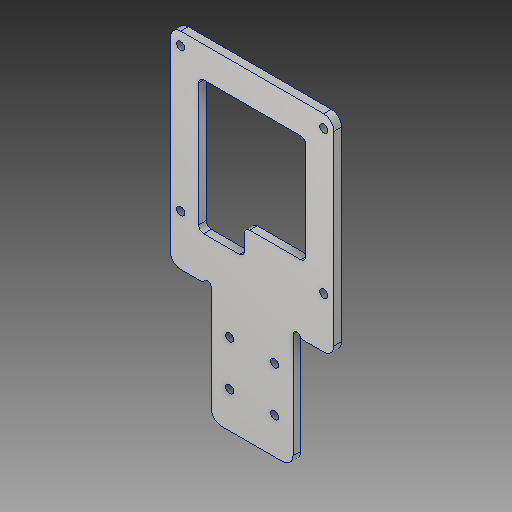
# Autodesk Inventor part: 手先カメラ
Saved by Autodesk Inventor 2017 (Build 210142000, 142)
## iProperties
Created: 2016-11-26
Part Number: 手先カメラ
Material: アルミニウム 6061
Document SubType Name: Modeling
Designer: NN
Density: 2.7 g/cm^3
Appearance: アルミニウム - フラット
Mass: 4.6771 g
Surface Area: 28.0851 cm^2
Volume: 1.73226 cm^3
Author: NN
Autodesk Inventor part; units mm, degrees
ref_plane "YZ Plane" through (0, 0, 0) normal (1, 0, 0) x (0, 1, 0)
ref_plane "XZ Plane" through (0, 0, 0) normal (0, 1, 0) x (-1, 0, 0)
ref_plane "XY Plane" through (0, 0, 0) normal (0, 0, 1) x (1, 0, 0)
sketch "スケッチ1" plane through (0, 0, 0) normal (0, 0, 1) x (1, 0, 0)
  line L0 (0, 0) -> (32, 0)
  line L1 (32, 0) -> (32, 63)
  line L2 (32, 63) -> (0, 63)
  line L3 (0, 63) -> (0, 0)
  dimension "d0" = 32
  dimension "d1" = 63
  constraints: 8 end point, 2 parallel, 1 horizontal, 1 perpendicular
  measures "d0" distance of L1.end L2.end
  measures "d1" distance between parallel lines of L0 L2
extrude "押し出し1" add sketch "スケッチ1" along normal blind 1.5
sketch "スケッチ2" plane through (0, 0, 1.5) normal (0, 0, 1) x (1, 0, 0)
  line L0 (2, 60.5) -> (30, 60.5)
  line L1 (30, 60.5) -> (30, 32.5)
  line L2 (30, 32.5) -> (2, 32.5)
  line L3 (2, 32.5) -> (2, 60.5)
  line L4 (32, 63) -> (0, 63) projected
  line L5 (16, 63) -> (16, 60.5)
  point P0 (0, 0)
  dimension "d4" = 28
  dimension "d5" = 28
  dimension "d6" = 2.5
  constraints: 10 end point, 2 midpoint, 2 parallel, 2 perpendicular, 1 horizontal
  measures "d4" distance of L0.start L0.end
  measures "d5" distance of L2.end L0.start
  measures "d6" distance between parallel lines of L4 L0
hole "穴1" at (30, 60.5, 1.5) at (2, 60.5, 1.5) at (30, 32.5, 1.5) at (2, 32.5, 1.5) direction (0, 0, -1) diameter 1.567 end through all thread size "M2x0.4" class "6H" standard "ISO Metric profile"
sketch "スケッチ3" plane through (0, 0, 1.5) normal (0, 0, 1) x (1, 0, 0)
  circle A0 centre (30, 32.5) radius 0.7835 projected
  circle A1 centre (30, 60.5) radius 0.7835 projected
  circle A2 centre (2, 60.5) radius 0.7835 projected
  circle A3 centre (2, 32.5) radius 0.7835 projected
  line L0 (0, 0) -> (32, 0) projected
  line L1 (32, 0) -> (32, 63) projected
  line L2 (32, 63) -> (0, 63) projected
  line L3 (0, 63) -> (0, 0) projected
  line L4 (0, 0) -> (8, 0)
  line L5 (8, 0) -> (8, 22.6)
  line L6 (8, 22.6) -> (0, 22.6)
  line L7 (0, 22.6) -> (0, 0)
  line L8 (0, 0) -> (32, 0) projected
  line L9 (16, 0) -> (16, 3.4564)
  line L10 (32, 0) -> (24, 0)
  line L11 (24, 0) -> (24, 22.6)
  line L12 (24, 22.6) -> (32, 22.6)
  line L13 (32, 22.6) -> (32, 0)
  dimension "d14" = 22.6
  dimension "d15" = 16
  constraints: 18 end point, 5 symmetric about line, 2 parallel, 1 horizontal, 1 midpoint, 1 perpendicular, 1 vertical
  measures "d14" distance between parallel lines of L0 L6
  measures "d15" distance between parallel lines of L11 L5
extrude "押し出し2" cut sketch "スケッチ3" against normal through all contours L3 L6 L5 L0 | L11 L12 L1 L0
sketch "スケッチ4" plane through (0, 0, 1.5) normal (0, 0, 1) x (1, 0, 0)
  line L0 (8, 22.6) -> (8, 0) projected
  line L1 (8, 0) -> (24, 0) projected
  line L2 (24, 0) -> (24, 22.6) projected
  line L3 (24, 22.6) -> (32, 22.6) projected
  line L4 (32, 22.6) -> (32, 63) projected
  line L5 (32, 63) -> (0, 63) projected
  line L6 (0, 63) -> (0, 22.6) projected
  line L7 (0, 22.6) -> (8, 22.6) projected
  circle A0 centre (30, 32.5) radius 0.7835 projected
  circle A1 centre (30, 60.5) radius 0.7835 projected
  circle A2 centre (2, 60.5) radius 0.7835 projected
  circle A3 centre (2, 32.5) radius 0.7835 projected
  line L8 (11.6, 15.9) -> (20.4, 15.9)
  line L9 (20.4, 15.9) -> (20.4, 7.1)
  line L10 (20.4, 7.1) -> (11.6, 7.1)
  line L11 (11.6, 7.1) -> (11.6, 15.9)
  line L12 (8, 0) -> (24, 0) projected
  line L13 (16, 0) -> (16, 7.1)
  line L14 (24, 0) -> (24, 22.6) projected
  line L15 (8, 0) -> (24, 0) projected
  point P0 (0, 0)
  dimension "d18" = 8.8
  dimension "d19" = 8.8
  dimension "d27" = 6.7
  constraints: 10 end point, 2 midpoint, 2 parallel, 2 perpendicular, 1 horizontal
  measures "d18" distance of L9.end L10.end
  measures "d19" distance of L8.end L9.end
  measures "d27" distance between parallel lines of L3 L8
hole "穴2" at (20.4, 15.9, 1.5) at (20.4, 7.1, 1.5) at (11.6, 7.1, 1.5) at (11.6, 15.9, 1.5) direction (0, 0, -1) diameter 1.567 end through all thread size "M2x0.4" class "6H" standard "ISO Metric profile"
sketch "スケッチ5" plane through (0, 0, 0) normal (0, 0, -1) x (-1, 0, 0)
  line L0 (-6, 34.6) -> (-14, 34.6) projected
  line L1 (-14, 34.6) -> (-14, 31.4) projected
  line L2 (-14, 31.4) -> (-6, 31.4) projected
  line L3 (-6, 31.4) -> (-6, 34.6) projected
  line L4 (-14.5, 35.1) -> (-5.5, 35.1)
  line L5 (-5.5, 35.1) -> (-5.5, 30.9)
  line L6 (-5.5, 30.9) -> (-14.5, 30.9)
  line L7 (-14.5, 30.9) -> (-14.5, 35.1)
  point P0 (0, 0)
  dimension "d28" = 0.5
  constraints: 8 end point, 3 other
  measures "d28" distance between parallel lines of L4 L0
extrude "押し出し3" cut sketch "スケッチ5" against normal through all contours L3 L2 L1 L0 | L4 L5 L6 L7
fillet "フィレット1" radius 2 6 edges at (32, 63, 0.75) (0, 63, 0.75) (0, 22.6, 0.75) (32, 22.6, 0.75) (8, 0, 0.75) (24, 0, 0.75)
sketch "スケッチ6" plane through (0, 0, 1.5) normal (0, 0, 1) x (1, 0, 0)
  line L0 (14.5, 35.1) -> (14.5, 30.9) projected
  line L1 (14.5, 30.9) -> (5.5, 30.9) projected
  line L2 (5.5, 30.9) -> (5.5, 35.1) projected
  line L3 (5.5, 35.1) -> (14.5, 35.1) projected
  circle A0 centre (11.6, 7.1) radius 0.7835 projected
  circle A1 centre (20.4, 15.9) radius 0.7835 projected
  circle A2 centre (20.4, 7.1) radius 0.7835 projected
  circle A3 centre (11.6, 15.9) radius 0.7835 projected
  arc A4 (22, 0) -> (24, 2) centre (22, 2) ccw projected
  line L4 (24, 2) -> (24, 22.6) projected
  line L5 (24, 22.6) -> (30, 22.6) projected
  arc A5 (30, 22.6) -> (32, 24.6) centre (30, 24.6) ccw projected
  line L6 (32, 24.6) -> (32, 61) projected
  arc A6 (32, 61) -> (30, 63) centre (30, 61) ccw projected
  line L7 (30, 63) -> (2, 63) projected
  arc A7 (2, 63) -> (0, 61) centre (2, 61) ccw projected
  line L8 (0, 61) -> (0, 24.6) projected
  arc A8 (0, 24.6) -> (2, 22.6) centre (2, 24.6) ccw projected
  line L9 (2, 22.6) -> (8, 22.6) projected
  line L10 (8, 22.6) -> (8, 2) projected
  arc A9 (8, 2) -> (10, 0) centre (10, 2) ccw projected
  line L11 (10, 0) -> (22, 0) projected
  circle A10 centre (30, 32.5) radius 0.7835 projected
  circle A11 centre (30, 60.5) radius 0.7835 projected
  circle A12 centre (2, 60.5) radius 0.7835 projected
  circle A13 centre (2, 32.5) radius 0.7835 projected
  line L12 (8, 22.6) -> (2, 22.6) projected
  circle A14 centre (7.25, 22.6) radius 0.75
  line L13 (30, 22.6) -> (24, 22.6) projected
  circle A15 centre (24.75, 22.6) radius 0.75
  line L14 (8, 22.6) -> (8, 2) projected
  line L15 (24, 2) -> (24, 22.6) projected
  point P0 (0, 0)
  dimension "d34" = 1.5
  dimension "d35" = 1.5
  constraints: 2 centre point, 2 point on line, 2 tangent
  measures "d34" diameter of A14
  measures "d35" diameter of A15
extrude "押し出し4" cut sketch "スケッチ6" against normal through all contours A15 L5 | L5 A15 | A14 L9 | L9 A14
fillet "フィレット2" radius 1 4 edges at (8, 22.6, 0.75) (6.5, 22.6, 0.75) (25.5, 22.6, 0.75) (24, 22.6, 0.75)
sketch "スケッチ7" plane through (0, 0, 1.5) normal (0, 0, 1) x (1, 0, 0)
  arc A0 (25.3655, 23.0286) -> (26.1861, 22.6) centre (26.1861, 23.6) ccw projected
  line L0 (26.1861, 22.6) -> (30, 22.6) projected
  arc A1 (30, 22.6) -> (32, 24.6) centre (30, 24.6) ccw projected
  line L1 (32, 24.6) -> (32, 61) projected
  arc A2 (32, 61) -> (30, 63) centre (30, 61) ccw projected
  line L2 (30, 63) -> (2, 63) projected
  arc A3 (2, 63) -> (0, 61) centre (2, 61) ccw projected
  line L3 (0, 61) -> (0, 24.6) projected
  arc A4 (0, 24.6) -> (2, 22.6) centre (2, 24.6) ccw projected
  line L4 (2, 22.6) -> (5.8139, 22.6) projected
  arc A5 (5.8139, 22.6) -> (6.6345, 23.0286) centre (5.8139, 23.6) ccw projected
  arc A6 (8, 22.6) -> (6.6345, 23.0286) centre (7.25, 22.6) ccw projected
  line L5 (8, 22.6) -> (8, 2) projected
  arc A7 (8, 2) -> (10, 0) centre (10, 2) ccw projected
  line L6 (10, 0) -> (22, 0) projected
  arc A8 (22, 0) -> (24, 2) centre (22, 2) ccw projected
  line L7 (24, 2) -> (24, 22.6) projected
  arc A9 (25.3655, 23.0286) -> (24, 22.6) centre (24.75, 22.6) ccw projected
  line L8 (14.5, 35.1) -> (14.5, 30.9) projected
  line L9 (14.5, 30.9) -> (5.5, 30.9) projected
  line L10 (5.5, 30.9) -> (5.5, 35.1) projected
  line L11 (5.5, 35.1) -> (14.5, 35.1) projected
  circle A10 centre (11.6, 7.1) radius 0.7835 projected
  circle A11 centre (20.4, 15.9) radius 0.7835 projected
  circle A12 centre (20.4, 7.1) radius 0.7835 projected
  circle A13 centre (11.6, 15.9) radius 0.7835 projected
  circle A14 centre (30, 32.5) radius 0.7835 projected
  circle A15 centre (30, 60.5) radius 0.7835 projected
  circle A16 centre (2, 60.5) radius 0.7835 projected
  circle A17 centre (2, 32.5) radius 0.7835 projected
  circle A18 centre (2, 60.5) radius 0.7835 projected
  line L12 (2, 60.5) -> (30, 60.5)
  line L13 (30, 60.5) -> (30, 32.5)
  line L14 (30, 32.5) -> (2, 32.5)
  line L15 (2, 32.5) -> (2, 60.5)
  line L16 (26.5, 57) -> (5.5, 57)
  line L17 (5.5, 57) -> (5.5, 36)
  line L18 (5.5, 36) -> (26.5, 36)
  line L19 (26.5, 36) -> (26.5, 57)
  point P0 (0, 0)
  dimension "d38" = 21
  constraints: 16 end point, 4 parallel, 2 perpendicular, 1 horizontal, 3 other
  measures "d38" distance between parallel lines of L19 L17
extrude "押し出し5" cut sketch "スケッチ7" against normal through all contours L19 L18 L17 L16
sketch "スケッチ8" plane through (0, 0, 1.5) normal (0, 0, 1) x (1, 0, 0)
  line L0 (5.5, 36) -> (5.5, 57) projected
  line L1 (5.5, 57) -> (26.5, 57) projected
  line L2 (26.5, 57) -> (26.5, 36) projected
  line L3 (26.5, 36) -> (5.5, 36) projected
  arc A0 (25.3655, 23.0286) -> (26.1861, 22.6) centre (26.1861, 23.6) ccw projected
  line L4 (26.1861, 22.6) -> (30, 22.6) projected
  arc A1 (30, 22.6) -> (32, 24.6) centre (30, 24.6) ccw projected
  line L5 (32, 24.6) -> (32, 61) projected
  arc A2 (32, 61) -> (30, 63) centre (30, 61) ccw projected
  line L6 (30, 63) -> (2, 63) projected
  arc A3 (2, 63) -> (0, 61) centre (2, 61) ccw projected
  line L7 (0, 61) -> (0, 24.6) projected
  arc A4 (0, 24.6) -> (2, 22.6) centre (2, 24.6) ccw projected
  line L8 (2, 22.6) -> (5.8139, 22.6) projected
  arc A5 (5.8139, 22.6) -> (6.6345, 23.0286) centre (5.8139, 23.6) ccw projected
  arc A6 (8, 22.6) -> (6.6345, 23.0286) centre (7.25, 22.6) ccw projected
  line L9 (8, 22.6) -> (8, 2) projected
  arc A7 (8, 2) -> (10, 0) centre (10, 2) ccw projected
  line L10 (10, 0) -> (22, 0) projected
  arc A8 (22, 0) -> (24, 2) centre (22, 2) ccw projected
  line L11 (24, 2) -> (24, 22.6) projected
  arc A9 (25.3655, 23.0286) -> (24, 22.6) centre (24.75, 22.6) ccw projected
  line L12 (14.5, 35.1) -> (14.5, 30.9) projected
  line L13 (14.5, 30.9) -> (5.5, 30.9) projected
  line L14 (5.5, 30.9) -> (5.5, 35.1) projected
  line L15 (5.5, 35.1) -> (14.5, 35.1) projected
  circle A10 centre (11.6, 7.1) radius 0.7835 projected
  circle A11 centre (20.4, 15.9) radius 0.7835 projected
  circle A12 centre (20.4, 7.1) radius 0.7835 projected
  circle A13 centre (11.6, 15.9) radius 0.7835 projected
  circle A14 centre (30, 32.5) radius 0.7835 projected
  circle A15 centre (30, 60.5) radius 0.7835 projected
  circle A16 centre (2, 60.5) radius 0.7835 projected
  circle A17 centre (2, 32.5) radius 0.7835 projected
  line L16 (5.5, 36) -> (5.5, 35.1)
  line L17 (14.5, 35.1) -> (14.5, 36)
  point P0 (0, 0)
  constraints: 4 end point, 1 perpendicular, 1 point on line, 1 vertical
extrude "押し出し6" cut sketch "スケッチ8" against normal through all contours L3 L17 L15 L16
fillet "フィレット5" radius 1 6 edges at (5.5, 57, 0.75) (26.5, 57, 0.75) (26.5, 36, 0.75) (14.5, 30.9, 0.75) (5.5, 30.9, 0.75) (14.5, 36, 0.75)
